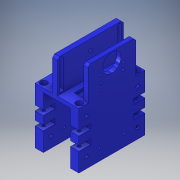
# Autodesk Inventor part: КВ33.044.501 - Каретка оси Y
Saved by Autodesk Inventor 2019 (Build 230136000, 136)
## iProperties
Created: 2019-07-21
Part Number: КВ33.044.501 - Каретка оси Y
Material: Пластик АБС
Document SubType Name: Modeling
Designer: Петров Иван
Density: 1.06 g/cm^3
Appearance: Синий — малярная краска — глянцевая
Mass: 139.056 g
Surface Area: 506.094 cm^2
Volume: 131.185 cm^3
Author: Петров Иван
Autodesk Inventor part; units mm, degrees
(part 1 of 2)
ref_plane "YZ Plane" through (0, 0, 0) normal (1, 0, 0) x (0, 1, 0)
ref_plane "XZ Plane" through (0, 0, 0) normal (0, 1, 0) x (-1, 0, 0)
ref_plane "XY Plane" through (0, 0, 0) normal (0, 0, 1) x (1, 0, 0)
sketch "Эскиз1" plane through (0, 0, 0) normal (1, 0, 0) x (0, 1, 0)
  line L0 (-34, 40) -> (34, 40)
  line L1 (34, 40) -> (34, -40)
  line L2 (34, -40) -> (-34, -40)
  line L3 (-34, -40) -> (-34, 40)
  line L4 (-34, 40) -> (34, -40) construction
  line L5 (34, 40) -> (-34, -40) construction
  line L6 (0, 0) -> (0, 31)
  line L7 (0, 31) -> (21.3, 31)
  line L8 (0, 31) -> (-21.3, 31)
  line L9 (0, 0) -> (0, -31)
  line L10 (0, -31) -> (21.3, -31)
  line L11 (0, -31) -> (-21.3, -31)
  circle A0 centre (21.3, 31) radius 2.1
  circle A1 centre (-21.3, 31) radius 2.1
  circle A2 centre (21.3, -31) radius 2.1
  circle A3 centre (-21.3, -31) radius 2.1
  dimension "d0" = 68
  dimension "d1" = 80
  dimension "d2" = 21.3
  dimension "d3" = 21.3
  dimension "d4" = 31
  dimension "d5" = 31
  dimension "d6" = 21.3
  dimension "d7" = 21.3
  dimension "d8" = 4.2
  dimension "d9" = 4.2
  dimension "d10" = 4.2
  dimension "d11" = 4.2
  constraints: 24 end point, 4 centre point, 4 coincident, 3 horizontal, 3 perpendicular, 2 midpoint, 2 parallel, 2 vertical
  measures "d0" distance of L1.end L2.end
  measures "d1" distance of L0.end L1.end
  measures "d2" distance of L6.end L7.end
  measures "d3" distance of L6.end L8.end
  measures "d4" distance of L6.start L6.end
  measures "d5" distance of L6.start L9.end
  measures "d6" distance of L9.end L10.end
  measures "d7" distance of L9.end L11.end
  measures "d8" diameter of A0
  measures "d9" diameter of A1
  measures "d10" diameter of A2
  measures "d11" diameter of A3
extrude "Выдавливание1" add sketch "Эскиз1" along normal blind 10
sketch "Эскиз2" plane through (10, 0, 0) normal (1, 0, 0) x (0, 0, -1)
  line L0 (-40, 34) -> (-40, -34) projected
  line L1 (-40, 0) -> (-40, 5)
  line L2 (-40, 0) -> (-26, 0)
  line L3 (-26, 0) -> (-26, 11)
  line L4 (-40, 5) -> (-26, 5)
  line L5 (-26, 5) -> (-26, 11)
  line L6 (-26, 11) -> (-40, 11)
  line L7 (-40, 11) -> (-40, 5)
  line L8 (-40, 0) -> (-40, -5)
  line L9 (-26, 0) -> (-26, -11)
  line L10 (-40, -5) -> (-26, -5)
  line L11 (-26, -5) -> (-26, -11)
  line L12 (-26, -11) -> (-40, -11)
  line L13 (-40, -11) -> (-40, -5)
  line L14 (40, -34) -> (40, 34) projected
  line L15 (40, 0) -> (40, 5)
  line L16 (40, 0) -> (26, 0)
  line L17 (26, 0) -> (26, 11)
  line L18 (26, 11) -> (40, 11)
  line L19 (40, 11) -> (40, 5)
  line L20 (40, 5) -> (26, 5)
  line L21 (26, 5) -> (26, 11)
  line L22 (26, 0) -> (26, -11)
  line L23 (40, 0) -> (40, -5)
  line L24 (26, -11) -> (40, -11)
  line L25 (40, -11) -> (40, -5)
  line L26 (40, -5) -> (26, -5)
  line L27 (26, -5) -> (26, -11)
  point P0 (0, 0)
  dimension "d14" = 5
  dimension "d15" = 14
  dimension "d16" = 11
  dimension "d17" = 5
  dimension "d18" = 11
  dimension "d19" = 5
  dimension "d20" = 14
  dimension "d21" = 11
  dimension "d22" = 11
  dimension "d23" = 5
  constraints: 52 end point, 8 parallel, 7 perpendicular, 5 horizontal, 4 point on line, 2 midpoint, 2 vertical
  measures "d14" distance of L1.start L1.end
  measures "d15" distance of L1.start L2.end
  measures "d16" distance of L2.end L3.end
  measures "d17" distance of L1.start L8.end
  measures "d18" distance of L2.end L9.end
  measures "d19" distance of L15.start L15.end
  measures "d20" distance of L15.start L16.end
  measures "d21" distance of L16.end L17.end
  measures "d22" distance of L16.end L22.end
  measures "d23" distance of L15.start L23.end
extrude "Выдавливание2" cut sketch "Эскиз2" against normal blind 10 contours L6 L3 L4 L0 | L10 L9 L12 L0 | L24 L22 L26 L14 | L20 L17 L18 L14
sketch "Эскиз3" plane through (0, 34, 40) normal (0, 1, 0) x (1, 0, 0)
  line L0 (0, 0) -> (10, 0) projected
  line L1 (5, 0) -> (5, 11.1)
  line L2 (0, 11.1) -> (10, 11.1) projected
  circle A0 centre (5, 5.55) radius 1.8
  line L3 (0, 80) -> (10, 80) projected
  line L4 (5, 80) -> (5, 68.9)
  line L5 (0, 68.9) -> (10, 68.9) projected
  circle A1 centre (5, 74.45) radius 1.8
  point P0 (0, 40)
  dimension "d26" = 3.6
  dimension "d29" = 3.6
  constraints: 6 midpoint, 4 end point, 2 centre point
  measures "d26" diameter of A0
  measures "d29" diameter of A1
extrude "Выдавливание3" cut sketch "Эскиз3" against normal through all
sketch "Эскиз4" plane through (0, 34, 40) normal (0, 1, 0) x (1, 0, 0)
  circle A0 centre (5, 5.55) radius 1.8 projected
  circle A1 centre (5, 5.55) radius 4
  circle A2 centre (5, 74.45) radius 1.8 projected
  circle A3 centre (5, 74.45) radius 4
  point P0 (0, 40)
  dimension "d30" = 8
  dimension "d31" = 8
  constraints: 2 centre point, 2 coincident
  measures "d30" diameter of A1
  measures "d31" diameter of A3
extrude "Выдавливание4" cut sketch "Эскиз4" against normal blind 10
sketch "Эскиз5" plane through (10, 0, 0) normal (1, 0, 0) x (0, 0, -1)
  line L0 (0, 0) -> (0, 18)
  line L1 (0, 18) -> (0, 20)
  line L2 (0, 20) -> (-15, 20)
  line L3 (-15, 20) -> (15, 20)
  circle A0 centre (-15, 20) radius 1.5
  circle A1 centre (15, 20) radius 1.5
  line L4 (0, 0) -> (6.6954, 0)
  line L5 (0, -18) -> (0, -20)
  line L6 (0, -20) -> (-15, -20)
  line L7 (-15, -20) -> (15, -20)
  circle A2 centre (-15, -20) radius 1.5
  circle A3 centre (15, -20) radius 1.5
  dimension "d34" = 18
  dimension "d35" = 2
  dimension "d36" = 15
  dimension "d37" = 30
  dimension "d38" = 3
  dimension "d39" = 3
  constraints: 16 end point, 6 symmetric about line, 4 centre point, 4 coincident, 3 point on line, 2 horizontal, 1 vertical, 2 other
  measures "d34" distance of L0.start L0.end
  measures "d35" distance of L0.end L1.end
  measures "d36" distance of L1.end L2.end
  measures "d37" distance of L2.end L3.end
  measures "d38" diameter of A0
  measures "d39" diameter of A1
extrude "Выдавливание5" cut sketch "Эскиз5" against normal blind 10 contours A2 | A3
sketch "Эскиз6" plane through (10, 0, 0) normal (1, 0, 0) x (0, 0, -1)
  circle A0 centre (15, -20) radius 1.5 projected
  circle A1 centre (-15, -20) radius 1.5 projected
  circle A2 centre (-31, 21.3) radius 2.1 projected
  circle A3 centre (-31, -21.3) radius 2.1 projected
  circle A4 centre (31, 21.3) radius 2.1 projected
  circle A5 centre (31, -21.3) radius 2.1 projected
  line L0 (-40, 11) -> (-26, 11) projected
  line L1 (-26, 11) -> (-26, 5) projected
  line L2 (-26, 5) -> (-40, 5) projected
  line L3 (-40, 5) -> (-40, -5) projected
  line L4 (-40, -5) -> (-26, -5) projected
  line L5 (-26, -5) -> (-26, -11) projected
  line L6 (-26, -11) -> (-40, -11) projected
  line L7 (-40, -11) -> (-40, -34) projected
  line L8 (-40, -34) -> (40, -34) projected
  line L9 (40, -34) -> (40, -11) projected
  line L10 (40, -11) -> (26, -11) projected
  line L11 (26, -11) -> (26, -5) projected
  line L12 (26, -5) -> (40, -5) projected
  line L13 (40, -5) -> (40, 5) projected
  line L14 (40, 5) -> (26, 5) projected
  line L15 (26, 5) -> (26, 11) projected
  line L16 (26, 11) -> (40, 11) projected
  line L17 (40, 11) -> (40, 34) projected
  line L18 (40, 34) -> (-40, 34) projected
  line L19 (-40, 34) -> (-40, 11) projected
  point P0 (0, 0)
sketch "Эскиз8" plane through (0, 0, 0) normal (-1, 0, 0) x (0, 0, 1)
  line L0 (-40, 34) -> (-40, 11) projected
  line L1 (40, 11) -> (40, 34) projected
  line L2 (-40, 34) -> (40, 34)
  line L3 (40, 34) -> (40, 29)
  line L4 (40, 29) -> (-40, 29)
  line L5 (-40, 29) -> (-40, 34)
  point P0 (0, 0)
  dimension "d46" = 5
  constraints: 8 end point, 2 parallel, 1 horizontal, 1 perpendicular, 1 point on line
  measures "d46" distance of L2.end L3.end
extrude "Выдавливание7" add sketch "Эскиз8" along normal blind 33
sketch "Эскиз13" plane through (-33, 0, 0) normal (-1, 0, 0) x (0, 0, 1)
  circle A0 centre (15, -20) radius 1.5
  circle A1 centre (-15, -20) radius 1.5
  circle A2 centre (-31, 21.3) radius 2.1
  circle A3 centre (-31, -21.3) radius 2.1
  circle A4 centre (31, 21.3) radius 2.1
  circle A5 centre (31, -21.3) radius 2.1
  line L0 (-40, 11) -> (-26, 11)
  line L1 (-26, 11) -> (-26, 5)
  line L2 (-26, 5) -> (-40, 5)
  line L3 (-40, 5) -> (-40, -5)
  line L4 (-40, -5) -> (-26, -5)
  line L5 (-26, -5) -> (-26, -11)
  line L6 (-26, -11) -> (-40, -11)
  line L7 (-40, -11) -> (-40, -34)
  line L8 (-40, -34) -> (40, -34)
  line L9 (40, -34) -> (40, -11)
  line L10 (40, -11) -> (26, -11)
  line L11 (26, -11) -> (26, -5)
  line L12 (26, -5) -> (40, -5)
  line L13 (40, -5) -> (40, 5)
  line L14 (40, 5) -> (26, 5)
  line L15 (26, 5) -> (26, 11)
  line L16 (26, 11) -> (40, 11)
  line L17 (40, 11) -> (40, 34)
  line L18 (40, 34) -> (-40, 34)
  line L19 (-40, 34) -> (-40, 11)
  point P0 (0, 0)
  point P1 (0, 0)
  constraints: 40 end point, 6 centre point
extrude "Выдавливание11" add sketch "Эскиз13" along normal blind 10
sketch "Эскиз14" plane through (10, 34, 40) normal (0, 1, 0) x (1, 0, 0)
  line L0 (0, 80) -> (-53, 80) projected
  line L1 (-26.5, 80) -> (-26.5, 69.4857)
  circle A0 centre (-5, 5.55) radius 4 projected
  circle A1 centre (-5, 74.45) radius 4 projected
  line L2 (0, 0) -> (-53, 0) projected
  line L3 (0, 80) -> (0, 0) projected
  line L4 (0, 80) -> (-53, 80) projected
  line L5 (-53, 0) -> (-53, 80) projected
  circle A2 centre (-5, 5.55) radius 1.8 projected
  circle A3 centre (-5, 74.45) radius 1.8 projected
  circle A4 centre (-48, 5.55) radius 1.8
  circle A5 centre (-48, 74.45) radius 1.8
  point P0 (-10, 40)
  constraints: 2 centre point, 2 end point, 2 symmetric about line, 1 midpoint, 1 vertical, 2 other
extrude "Выдавливание12" cut sketch "Эскиз14" against normal through all contours A4 | A5
sketch "Эскиз15" plane through (10, 34, 40) normal (0, 1, 0) x (1, 0, 0)
  circle A0 centre (-48, 74.45) radius 1.8 projected
  circle A1 centre (-48, 74.45) radius 4
  circle A2 centre (-48, 5.55) radius 1.8 projected
  circle A3 centre (-48, 5.55) radius 4
  point P0 (-10, 40)
  dimension "d65" = 8
  dimension "d66" = 8
  constraints: 2 centre point, 2 coincident
  measures "d65" diameter of A1
  measures "d66" diameter of A3
extrude "Выдавливание13" cut sketch "Эскиз15" against normal blind 20
sketch "Эскиз16" plane through (10, 34, 40) normal (0, 1, 0) x (1, 0, 0)
  circle A0 centre (-48, 74.45) radius 4 projected
  circle A1 centre (-48, 5.55) radius 4 projected
  circle A2 centre (-5, 5.55) radius 4 projected
  circle A3 centre (-5, 74.45) radius 4 projected
  line L0 (0, 0) -> (-53, 0) projected
  line L1 (0, 80) -> (0, 0) projected
  line L2 (0, 80) -> (-53, 80) projected
  line L3 (-53, 0) -> (-53, 80) projected
  point P0 (-10, 40)
sketch "Эскиз17" plane through (-33, -34, -40) normal (0, -1, 0) x (1, 0, 0)
  circle A0 centre (-5, 5.55) radius 4
  circle A1 centre (-5, 74.45) radius 4
  circle A2 centre (-5, 5.55) radius 1.8 projected
  line L0 (-5, 5.55) -> (-5, 18.1127)
  circle A3 centre (38, 74.45) radius 4
  circle A4 centre (38, 5.55) radius 4
  circle A5 centre (-5, 5.55) radius 4
  circle A6 centre (-5, 74.45) radius 4
  line L1 (-10, 0) -> (43, 0)
  line L2 (-10, 80) -> (-10, 0)
  line L3 (-10, 80) -> (43, 80)
  line L4 (43, 0) -> (43, 80)
  circle A7 centre (-5, 5.55) radius 1.8
  point P0 (33, 40)
  point P1 (-10, 40)
  point P2 (0, 40)
  constraints: 10 end point, 7 centre point, 1 symmetric about line, 1 vertical, 3 other
extrude "Выдавливание14" cut sketch "Эскиз17" against normal blind 20 contours A0 | A1 | A3 | A4
sketch "Эскиз25" plane through (10, 34, 40) normal (0, 1, 0) x (1, 0, 0)
  line L0 (-10, 68.9) -> (0, 68.9) projected
  line L1 (-10, 11.1) -> (0, 11.1) projected
  line L2 (-5, 68.9) -> (0, 68.9)
  line L3 (0, 68.9) -> (0, 11.1)
  line L4 (0, 11.1) -> (-5, 11.1)
  line L5 (-5, 11.1) -> (-5, 68.9)
  point P0 (-10, 40)
  constraints: 8 end point, 2 parallel, 1 horizontal, 1 midpoint, 1 perpendicular, 1 point on line
extrude "Выдавливание21" add sketch "Эскиз25" along normal blind 40
sketch "Эскиз26" plane through (10, 0, 0) normal (1, 0, 0) x (0, 0, -1)
  line L0 (-12.6, 44.2) -> (-14.9, 44.2)
  line L1 (-12.6, 44.2) -> (-12.6, 42.8)
  line L2 (-14.9, 42.8) -> (-12.6, 42.8)
  line L3 (-14.9, 36.2) -> (-14.9, 42.8)
  line L4 (-12.6, 36.2) -> (-14.9, 36.2)
  circle A0 centre (0, 62) radius 9.15
  circle A1 centre (0, 62) radius 1.5
  circle A2 centre (8, 26) radius 1.3
  circle A3 centre (13.5, 39.5) radius 1.3
  circle A4 centre (13.5, 31.5) radius 1.3
  circle A5 centre (13.5, 47.5) radius 1.3
  circle A6 centre (13.5, 55.5) radius 1.3
  circle A7 centre (-8, 26) radius 1.3
  circle A8 centre (-13.5, 39.5) radius 1.3
  circle A9 centre (-13.5, 31.5) radius 1.3
  circle A10 centre (-13.5, 47.5) radius 1.3
  circle A11 centre (-13.5, 55.5) radius 1.3
  line L5 (-0.1, 73.0198) -> (-0.1, 72.4796)
  line L6 (-7, 73.0198) -> (-0.1, 73.0198)
  arc A12 (-7, 73.0198) -> (-7.75, 72.9686) centre (-7, 67.5) ccw
  line L7 (-7.75, 70.5) -> (-7.75, 72.9686)
  arc A13 (-9.5, 68.75) -> (-7.75, 70.5) centre (-9.5, 70.5) ccw
  line L8 (-10, 68.75) -> (-9.5, 68.75)
  line L9 (-10, 31.1937) -> (-10, 68.75)
  arc A14 (-10, 31.1937) -> (-9.6078, 30.5055) centre (-9.2, 31.1937) ccw
  arc A15 (-9.6078, 30.5055) -> (-8.9945, 29.8922) centre (-10.5, 29) ccw
  arc A16 (-8.9945, 29.8922) -> (-8.3063, 29.5) centre (-8.3063, 30.3) ccw
  line L10 (8.3063, 29.5) -> (-8.3063, 29.5)
  arc A17 (8.3063, 29.5) -> (8.9945, 29.8922) centre (8.3063, 30.3) ccw
  arc A18 (9.6078, 30.5055) -> (8.9945, 29.8922) centre (10.5, 29) ccw
  arc A19 (8.9945, 29.8922) -> (9.6078, 30.5055) centre (10.5, 29) ccw
  line L11 (-11.3229, 68.75) -> (-10, 68.75)
  arc A20 (-11.3229, 68.75) -> (-11.5, 67.4989) centre (-6.9922, 67.4989) ccw
  line L12 (-11.5, 67.4989) -> (-11.5, 60)
  line L13 (-12.6, 60) -> (-11.5, 60)
  line L14 (-12.6, 58.8) -> (-12.6, 60)
  line L15 (-14.9, 58.8) -> (-12.6, 58.8)
  line L16 (-14.9, 52.2) -> (-14.9, 58.8)
  line L17 (-12.6, 52.2) -> (-14.9, 52.2)
  line L18 (-12.6, 50.8) -> (-12.6, 52.2)
  line L19 (-14.9, 50.8) -> (-12.6, 50.8)
  line L20 (-14.9, 44.2) -> (-14.9, 50.8)
  line L21 (-12.6, 44.2) -> (-14.9, 44.2)
  line L22 (-12.6, 42.8) -> (-12.6, 44.2)
  line L23 (-14.9, 42.8) -> (-12.6, 42.8)
  line L24 (-14.9, 36.2) -> (-14.9, 42.8)
  line L25 (-12.6, 36.2) -> (-14.9, 36.2)
  line L26 (-12.6, 34.8) -> (-12.6, 36.2)
  line L27 (-14.9, 34.8) -> (-12.6, 34.8)
  line L28 (-14.9, 28.2) -> (-14.9, 34.8)
  line L29 (-12.6, 28.2) -> (-14.9, 28.2)
  line L30 (-12.6, 26.9802) -> (-12.6, 28.2)
  arc A21 (-12.6, 26.9802) -> (-12.5198, 26.9) centre (-11.5, 28) ccw
  line L31 (-11.3, 26.9) -> (-12.5198, 26.9)
  line L32 (-11.3, 24.6) -> (-11.3, 26.9)
  line L33 (-4.7, 24.6) -> (-11.3, 24.6)
  line L34 (-4.7, 26.9) -> (-4.7, 24.6)
  line L35 (4.7, 26.9) -> (-4.7, 26.9)
  line L36 (4.7, 24.6) -> (4.7, 26.9)
  line L37 (11.3, 24.6) -> (4.7, 24.6)
  line L38 (11.3, 26.9) -> (11.3, 24.6)
  line L39 (12.5198, 26.9) -> (11.3, 26.9)
  arc A22 (12.5198, 26.9) -> (12.6, 26.9802) centre (11.5, 28) ccw
  line L40 (12.6, 28.2) -> (12.6, 26.9802)
  line L41 (14.9, 28.2) -> (12.6, 28.2)
  line L42 (14.9, 34.8) -> (14.9, 28.2)
  line L43 (12.6, 34.8) -> (14.9, 34.8)
  line L44 (12.6, 36.2) -> (12.6, 34.8)
  line L45 (14.9, 36.2) -> (12.6, 36.2)
  line L46 (14.9, 42.8) -> (14.9, 36.2)
  line L47 (12.6, 42.8) -> (14.9, 42.8)
  line L48 (12.6, 44.2) -> (12.6, 42.8)
  line L49 (14.9, 44.2) -> (12.6, 44.2)
  line L50 (14.9, 50.8) -> (14.9, 44.2)
  line L51 (12.6, 50.8) -> (14.9, 50.8)
  line L52 (12.6, 52.2) -> (12.6, 50.8)
  line L53 (14.9, 52.2) -> (12.6, 52.2)
  line L54 (14.9, 58.8) -> (14.9, 52.2)
  line L55 (12.6, 58.8) -> (14.9, 58.8)
  line L56 (12.6, 60) -> (12.6, 58.8)
  line L57 (11.5, 60) -> (12.6, 60)
  line L58 (11.5, 67.5) -> (11.5, 60)
  arc A23 (11.5, 67.5) -> (11.3229, 68.75) centre (6.9922, 67.4989) ccw
  line L59 (10, 68.75) -> (11.3229, 68.75)
  line L60 (9.5, 68.75) -> (10, 68.75)
  arc A24 (7.75, 70.5) -> (9.5, 68.75) centre (9.5, 70.5) ccw
  line L61 (7.75, 72.9686) -> (7.75, 70.5)
  arc A25 (7.75, 72.9686) -> (7, 73.0198) centre (7, 67.5) ccw
  line L62 (0.1, 73.0198) -> (7, 73.0198)
  line L63 (0.1, 72.4796) -> (0.1, 73.0198)
  arc A26 (-8.9945, 29.8922) -> (-9.6078, 30.5055) centre (-10.5, 29) ccw
  arc A27 (9.6078, 30.5055) -> (10, 31.1895) centre (9.2, 31.1937) ccw
  line L64 (10, 68.75) -> (10, 31.1895)
  line L65 (0, 0) -> (0, 74)
  line L66 (28.9, 74) -> (-28.9, 74) projected
  line L67 (0, 74) -> (0, 62)
  point P0 (0, 62)
  dimension "d102" = 12
  constraints: 134 end point, 32 point on circle, 28 centre point, 1 midpoint, 1 point on line
  measures "d102" distance of L65.end L67.end
extrude "Выдавливание22" cut sketch "Эскиз26" against normal blind 40 contours A0 L65 A1 | L65 A1 A0 | L65 A1 | A1 L65 | A3 | A5 | A6 | A8 | A10 | A11
sketch "Эскиз29" plane through (-43, 34, -40) normal (0, 1, 0) x (1, 0, 0)
  line L0 (43, -11.1) -> (53, -11.1) projected
  line L1 (48, -11.1) -> (48, -68.9) projected
  line L2 (48, -11.1) -> (48, -68.9)
  circle A0 centre (40.9968, -58.9777) radius 1.5
  line L3 (33.923, -34.3302) -> (33.923, -66.4777)
  line L4 (33.923, -66.4777) -> (47.9968, -66.4777)
  line L5 (47.9968, -66.4777) -> (47.9968, -34.3302)
  line L6 (47.9968, -34.3302) -> (33.923, -34.3302)
  point P0 (43, -40)
  point P1 (40.9968, -50.4777)
  constraints: 10 end point, 1 centre point, 1 collinear, 1 midpoint
extrude "Выдавливание23" cut sketch "Эскиз29" against normal blind 4 contours A0 | L6 L5 L4 L3
sketch "Эскиз30" plane through (-43, 34, -40) normal (0, 1, 0) x (1, 0, 0)
  line L0 (43, -11.1) -> (53, -11.1) projected
  line L1 (48, -11.1) -> (28.26, -11.1)
  line L2 (43, 0) -> (10, 0) projected
  line L3 (53, -80) -> (0, -80) projected
  line L4 (27, 0) -> (21, 0)
  line L5 (21, 0) -> (21, -80)
  line L6 (21, -80) -> (27, -80)
  line L7 (27, -80) -> (27, 0)
  line L8 (48, -11.1) -> (48, -68.9) projected
  point P0 (43, -40)
  dimension "d115" = 19.74
  dimension "d116" = 6
  dimension "d119" = 21
  constraints: 10 end point, 2 parallel, 2 point on line, 1 collinear, 1 horizontal, 1 midpoint, 1 perpendicular
  measures "d115" distance of L1.start L1.end
  measures "d116" distance of L6.end L5.end
  measures "d119" distance between parallel lines of L8 L7
extrude "Выдавливание24" add sketch "Эскиз30" along normal blind 40
sketch "Эскиз31" plane through (-22, 34, -40) normal (-1, 0, 0) x (0, 0, 1)
  circle A0 centre (40, 28) radius 9.15 projected
  circle A1 centre (40, 28) radius 2
  point P0 (40, -34)
  dimension "d120" = 4
  constraints: 1 centre point, 1 coincident
  measures "d120" diameter of A1
extrude "Выдавливание25" cut sketch "Эскиз31" against normal blind 40 contours A1
sketch "Эскиз32" plane through (-16, 34, 40) normal (1, 0, 0) x (0, 0, -1)
  line L0 (0, 0) -> (0, 40) projected
  line L1 (0, 20) -> (5, 20)
  line L2 (5, 3.4608) -> (5, 36.5392) construction
  line L3 (7.1, 3.4608) -> (7.1, 36.5392)
  line L4 (2.9, 36.5392) -> (2.9, 3.4608)
  arc A0 (2.9, 3.4608) -> (7.1, 3.4608) centre (5, 3.4608) ccw
  arc A1 (7.1, 36.5392) -> (2.9, 36.5392) centre (5, 36.5392) ccw
  line L5 (80, 40) -> (0, 40) projected
  line L6 (40, 40) -> (40, 35.6564)
  line L7 (80, 20) -> (75, 20)
  line L8 (75, 3.4608) -> (75, 36.5392) construction
  line L9 (72.9, 3.4608) -> (72.9, 36.5392)
  line L10 (77.1, 36.5392) -> (77.1, 3.4608)
  arc A2 (72.9, 3.4608) -> (77.1, 3.4608) centre (75, 3.4608) ccw
  arc A3 (77.1, 36.5392) -> (72.9, 36.5392) centre (75, 36.5392) ccw
  point P0 (40, -34)
  dimension "d123" = 5
  dimension "d124" = 4.2
  constraints: 22 end point, 8 point on circle, 8 symmetric about line, 4 centre point, 4 tangent, 3 midpoint, 1 horizontal, 1 parallel, 1 perpendicular, 1 vertical, 2 other
  measures "d123" distance of L1.start L1.end
  measures "d124" diameter of A1
extrude "Выдавливание26" cut sketch "Эскиз32" against normal blind 40
sketch "Эскиз33" plane through (10, 0, 0) normal (1, 0, 0) x (0, 0, -1)
  circle A0 centre (0, 62) radius 2 projected
  circle A1 centre (0, 62) radius 11
  point P0 (0, 0)
  dimension "d127" = 22
  constraints: 1 centre point, 1 coincident
  measures "d127" diameter of A1
extrude "Выдавливание27" cut sketch "Эскиз33" against normal blind 6
chamfer "Фаска5" distance 2.75 angle 45 4 edges at (7.5, 74, 28.9) (7.5, 74, -28.9) (-19, 74, 40) (-19, 74, -40)
sketch "Эскиз43" plane through (-43, 34, 40) normal (0, 1, 0) x (1, 0, 0)
  line L0 (0.0943, 0) -> (0.6069, 0)
  line L1 (0.6069, 0) -> (0.6986, 1.434)
  arc A0 (4.89, 1.434) -> (0.6986, 1.434) centre (2.7943, 1.3) ccw
  line L2 (4.89, 1.434) -> (4.9817, 0)
  line L3 (4.9817, 0) -> (9.27, 0)
  arc A1 (9.27, 0) -> (9.3408, 0.0293) centre (9.27, 0.1) ccw
  line L4 (9.3408, 0.0293) -> (9.665, 0.3536)
  arc A2 (10.0186, 0.5) -> (9.665, 0.3536) centre (10.0186, 0) ccw
  line L5 (10.0186, 0.5) -> (19.6943, 0.5)
  arc A3 (19.6943, 0.5) -> (19.7943, 0.6) centre (19.6943, 0.6) ccw
  line L6 (19.7943, 0.6) -> (19.7943, 9.6674)
  arc A4 (19.7943, 9.6674) -> (19.6117, 9.85) centre (19.6943, 9.75) ccw
  line L7 (19.6117, 9.85) -> (16.7686, 9.85)
  arc A5 (16.415, 9.9965) -> (16.7686, 9.85) centre (16.7686, 10.35) ccw
  line L8 (16.415, 9.9965) -> (16.0908, 10.3207)
  arc A6 (16.0908, 10.3207) -> (16.02, 10.35) centre (16.02, 10.25) ccw
  line L9 (16.02, 10.35) -> (13.2686, 10.35)
  arc A7 (13.2686, 10.35) -> (13.1979, 10.3207) centre (13.2686, 10.25) ccw
  line L10 (13.1979, 10.3207) -> (12.8736, 9.9965)
  arc A8 (12.52, 9.85) -> (12.8736, 9.9965) centre (12.52, 10.35) ccw
  line L11 (12.52, 9.85) -> (7.2686, 9.85)
  arc A9 (6.915, 9.9965) -> (7.2686, 9.85) centre (7.2686, 10.35) ccw
  line L12 (6.915, 9.9965) -> (6.5908, 10.3207)
  arc A10 (6.5908, 10.3207) -> (6.52, 10.35) centre (6.52, 10.25) ccw
  line L13 (6.52, 10.35) -> (3.7686, 10.35)
  arc A11 (3.7686, 10.35) -> (3.6979, 10.3207) centre (3.7686, 10.25) ccw
  line L14 (3.6979, 10.3207) -> (3.3736, 9.9965)
  arc A12 (3.02, 9.85) -> (3.3736, 9.9965) centre (3.02, 10.35) ccw
  line L15 (3.02, 9.85) -> (0.0943, 9.85)
  arc A13 (0.0943, 9.85) -> (-0.0057, 9.75) centre (0.0943, 9.75) ccw
  line L16 (-0.0057, 9.75) -> (-0.0057, 0.1)
  arc A14 (-0.0057, 0.1) -> (0.0943, 0) centre (0.0943, 0.1) ccw
  circle A15 centre (5.1443, 7.8) radius 1.25
  circle A16 centre (14.6443, 7.8) radius 1.25
  line L17 (15.8176, 5.55) -> (15.201, 4.25)
  line L18 (15.201, 4.25) -> (15.1843, 4.25)
  line L19 (15.1843, 4.25) -> (14.5843, 5.55)
  line L20 (14.5843, 5.55) -> (14.7111, 5.55)
  line L21 (14.7111, 5.55) -> (14.9033, 5.1334)
  line L22 (14.9033, 5.1334) -> (15.4926, 5.1334)
  line L23 (15.4926, 5.1334) -> (15.6903, 5.55)
  line L24 (15.6903, 5.55) -> (15.8176, 5.55)
  spline S0 degree 3 poles (12.9976, 4.6136) (12.9979, 4.6047) (12.9983, 4.5872) (13.0025, 4.5616) (13.0087, 4.5369) (13.0176, 4.513) (13.0293, 4.4901) (13.0436, 4.4684) (13.0601, 4.4473) (13.0791, 4.4276) (13.1001, 4.4095) (13.1222, 4.3935) (13.1457, 4.3801) (13.1703, 4.3691) (13.196, 4.3605) (13.2229, 4.3545) (13.2508, 4.3508) (13.2699, 4.3503) (13.2797, 4.35) knots 0 0 0 0 0.061965 0.122122 0.180988 0.239933 0.299906 0.359989 0.421776 0.486576 0.551535 0.615018 0.677259 0.73973 0.80305 0.866495 0.931973 1 1 1 1
  spline S1 degree 3 poles (13.2797, 4.35) (13.2898, 4.3503) (13.3098, 4.3508) (13.3391, 4.3545) (13.3671, 4.3607) (13.3938, 4.3694) (13.4192, 4.3803) (13.4433, 4.3939) (13.466, 4.4102) (13.4873, 4.4286) (13.5069, 4.4492) (13.5242, 4.472) (13.5393, 4.4969) (13.5524, 4.5236) (13.5631, 4.5524) (13.5713, 4.5832) (13.5777, 4.6159) (13.5799, 4.6384) (13.581, 4.65) knots 0 0 0 0 0.064439 0.126547 0.186887 0.245878 0.304041 0.362191 0.420976 0.48066 0.5406 0.600689 0.661936 0.724443 0.789038 0.856314 0.926352 1 1 1 1
  line L25 (13.581, 4.65) -> (13.6976, 4.65)
  spline S2 degree 3 poles (13.6976, 4.65) (13.6969, 4.6345) (13.6954, 4.6041) (13.6884, 4.5598) (13.6784, 4.5175) (13.6642, 4.4774) (13.6467, 4.4393) (13.6256, 4.4032) (13.6006, 4.3694) (13.5723, 4.3382) (13.5416, 4.3095) (13.5084, 4.2848) (13.4736, 4.2638) (13.4371, 4.2464) (13.3987, 4.2332) (13.3586, 4.2235) (13.3167, 4.2176) (13.2882, 4.217) (13.2737, 4.2167) knots 0 0 0 0 0.068791 0.135103 0.198979 0.261904 0.323495 0.385195 0.446969 0.509765 0.572251 0.633405 0.693251 0.752583 0.812579 0.873275 0.93555 1 1 1 1
  spline S3 degree 3 poles (13.2737, 4.2167) (13.2594, 4.217) (13.2314, 4.2177) (13.1905, 4.2233) (13.1516, 4.2321) (13.1147, 4.2445) (13.0802, 4.2611) (13.0477, 4.2811) (13.0169, 4.3042) (12.9892, 4.3314) (12.9638, 4.3605) (12.9418, 4.3915) (12.923, 4.4235) (12.9074, 4.4568) (12.8958, 4.4917) (12.8871, 4.5276) (12.8821, 4.565) (12.8814, 4.5903) (12.881, 4.6031) knots 0 0 0 0 0.069475 0.136517 0.200789 0.26383 0.325735 0.387291 0.449509 0.512968 0.576275 0.63758 0.697903 0.757172 0.816599 0.876653 0.93729 1 1 1 1
  spline S4 degree 3 poles (12.881, 4.6031) (12.8816, 4.6213) (12.8829, 4.6571) (12.8935, 4.7099) (12.9102, 4.761) (12.9302, 4.8021) (12.9505, 4.8353) (12.9687, 4.8626) (12.99, 4.8919) (13.0148, 4.9233) (13.0425, 4.9569) (13.0733, 4.9928) (13.1075, 5.0305) (13.1316, 5.0562) (13.144, 5.0696) knots 0 0 0 0 0.098702 0.195672 0.292422 0.391343 0.444462 0.504229 0.570352 0.642546 0.722288 0.807921 0.90047 1 1 1 1
  line L26 (13.144, 5.0696) -> (13.4693, 5.4167)
  line L27 (13.4693, 5.4167) -> (12.8643, 5.4167)
  line L28 (12.8643, 5.4167) -> (12.8643, 5.55)
  line L29 (12.8643, 5.55) -> (13.7476, 5.55)
  line L30 (13.7476, 5.55) -> (13.2435, 5.012)
  spline S5 degree 3 poles (13.2435, 5.012) (13.2312, 4.9992) (13.2076, 4.9746) (13.1743, 4.9386) (13.1443, 4.9053) (13.1176, 4.8746) (13.0946, 4.8462) (13.0742, 4.8208) (13.0579, 4.7975) (13.0402, 4.7705) (13.023, 4.7375) (13.0083, 4.6972) (12.9993, 4.6557) (12.9982, 4.6277) (12.9976, 4.6136) knots 0 0 0 0 0.110803 0.212829 0.306101 0.390647 0.466924 0.534481 0.593587 0.644557 0.7362 0.825024 0.911986 1 1 1 1
  line L31 (12.4876, 4.9) -> (12.3543, 4.25)
  line L32 (12.3543, 4.25) -> (11.821, 4.25)
  line L33 (11.821, 4.25) -> (11.821, 4.3834)
  line L34 (11.821, 4.3834) -> (12.2632, 4.3834)
  line L35 (12.2632, 4.3834) -> (12.3332, 4.7253)
  spline S6 degree 3 poles (12.3332, 4.7253) (12.3195, 4.7215) (12.2928, 4.7141) (12.2534, 4.7059) (12.2161, 4.701) (12.1918, 4.7003) (12.1801, 4.7) knots 0 0 0 0 0.275068 0.532901 0.773973 1 1 1 1
  spline S7 degree 3 poles (12.1801, 4.7) (12.1656, 4.7003) (12.137, 4.701) (12.0953, 4.7069) (12.0554, 4.7162) (12.0175, 4.7293) (11.9815, 4.7459) (11.9478, 4.7668) (11.9158, 4.7911) (11.8861, 4.8191) (11.8592, 4.8499) (11.8355, 4.883) (11.8154, 4.9181) (11.7992, 4.9556) (11.7863, 4.9949) (11.7777, 5.0366) (11.7719, 5.0802) (11.7713, 5.1101) (11.771, 5.1253) knots 0 0 0 0 0.065808 0.129394 0.190894 0.251281 0.310815 0.370371 0.430768 0.492881 0.555104 0.616067 0.677256 0.73826 0.800762 0.864778 0.931045 1 1 1 1
  spline S8 degree 3 poles (11.771, 5.1253) (11.7712, 5.1359) (11.7717, 5.1569) (11.7742, 5.1882) (11.779, 5.2188) (11.7855, 5.2487) (11.7938, 5.2779) (11.804, 5.3065) (11.8164, 5.3343) (11.83, 5.3615) (11.8453, 5.3876) (11.8623, 5.412) (11.8803, 5.435) (11.8996, 5.4565) (11.9205, 5.4763) (11.9426, 5.4945) (11.9659, 5.5114) (11.9907, 5.5263) (12.0164, 5.54) (12.0433, 5.5513) (12.071, 5.5614) (12.0997, 5.5694) (12.1295, 5.5757) (12.1603, 5.5799) (12.192, 5.5831) (12.2135, 5.5833) (12.2244, 5.5834) knots 0 0 0 0 0.044014 0.087434 0.130118 0.172554 0.214555 0.256298 0.298438 0.340849 0.382715 0.423924 0.464246 0.504074 0.543862 0.583567 0.623094 0.663229 0.703551 0.743938 0.784541 0.82575 0.867757 0.910745 0.954914 1 1 1 1
  spline S9 degree 3 poles (12.2244, 5.5834) (12.2373, 5.5831) (12.2628, 5.5826) (12.3001, 5.5773) (12.3361, 5.5697) (12.3703, 5.5584) (12.4031, 5.5441) (12.4341, 5.5261) (12.464, 5.5057) (12.4917, 5.4816) (12.5174, 5.4552) (12.5404, 5.4266) (12.5609, 5.3963) (12.5785, 5.364) (12.5935, 5.3299) (12.6054, 5.2938) (12.6149, 5.256) (12.6189, 5.2299) (12.621, 5.2167) knots 0 0 0 0 0.065421 0.128708 0.190236 0.250724 0.310637 0.370766 0.431615 0.493523 0.555883 0.617342 0.678668 0.740711 0.802985 0.866803 0.932347 1 1 1 1
  line L36 (12.621, 5.2167) -> (12.5043, 5.2167)
  spline S10 degree 3 poles (12.5043, 5.2167) (12.5014, 5.2291) (12.4959, 5.2529) (12.4838, 5.2864) (12.469, 5.3162) (12.4514, 5.3428) (12.4304, 5.366) (12.4064, 5.3866) (12.3796, 5.4053) (12.3497, 5.4208) (12.3182, 5.4341) (12.2852, 5.4429) (12.2517, 5.4491) (12.229, 5.4497) (12.2176, 5.45) knots 0 0 0 0 0.094687 0.181994 0.264377 0.34218 0.418618 0.496509 0.577369 0.661511 0.746733 0.831258 0.915206 1 1 1 1
  spline S11 degree 3 poles (12.2176, 5.45) (12.2065, 5.4497) (12.1846, 5.4491) (12.1523, 5.4445) (12.1212, 5.4374) (12.0915, 5.4267) (12.0627, 5.4138) (12.0355, 5.3972) (12.0091, 5.3781) (11.9845, 5.3562) (11.9619, 5.332) (11.9419, 5.3062) (11.9253, 5.2787) (11.9113, 5.2499) (11.9006, 5.2196) (11.893, 5.1878) (11.8886, 5.1546) (11.888, 5.1319) (11.8876, 5.1203) knots 0 0 0 0 0.064207 0.126425 0.18768 0.248216 0.308305 0.369661 0.431699 0.495947 0.559758 0.622295 0.683911 0.745092 0.80674 0.869087 0.93329 1 1 1 1
  spline S12 degree 3 poles (11.8876, 5.1203) (11.8879, 5.1099) (11.8884, 5.0895) (11.8923, 5.0596) (11.8991, 5.0314) (11.9085, 5.0046) (11.9205, 4.9792) (11.9352, 4.9553) (11.9528, 4.9331) (11.9728, 4.9127) (11.9949, 4.8938) (12.0192, 4.8777) (12.0453, 4.8641) (12.0728, 4.8525) (12.1025, 4.8441) (12.1338, 4.8378) (12.1669, 4.8341) (12.1895, 4.8336) (12.2012, 4.8334) knots 0 0 0 0 0.065351 0.127916 0.18836 0.247216 0.30563 0.36377 0.422661 0.482687 0.5433 0.604118 0.664965 0.727413 0.791468 0.858055 0.927037 1 1 1 1
  spline S13 degree 3 poles (12.2012, 4.8334) (12.2113, 4.8336) (12.2321, 4.834) (12.264, 4.8373) (12.2975, 4.8426) (12.3325, 4.8499) (12.3692, 4.8594) (12.4073, 4.8708) (12.4471, 4.8844) (12.4739, 4.8947) (12.4876, 4.9) knots 0 0 0 0 0.102203 0.211023 0.3251 0.446502 0.573788 0.708901 0.850358 1 1 1 1
  line L37 (9.041, 5.55) -> (8.4243, 4.25)
  line L38 (8.4243, 4.25) -> (8.4076, 4.25)
  line L39 (8.4076, 4.25) -> (7.8076, 5.55)
  line L40 (7.8076, 5.55) -> (7.9345, 5.55)
  line L41 (7.9345, 5.55) -> (8.1267, 5.1334)
  line L42 (8.1267, 5.1334) -> (8.716, 5.1334)
  line L43 (8.716, 5.1334) -> (8.9136, 5.55)
  line L44 (8.9136, 5.55) -> (9.041, 5.55)
  spline S14 degree 3 poles (7.531, 4.8925) (7.5304, 4.8691) (7.5293, 4.8231) (7.5196, 4.7556) (7.5041, 4.6909) (7.482, 4.6291) (7.454, 4.57) (7.4195, 4.514) (7.3788, 4.4607) (7.3322, 4.4109) (7.2811, 4.3654) (7.2263, 4.3254) (7.1681, 4.292) (7.107, 4.2642) (7.0426, 4.2428) (6.9749, 4.2278) (6.9042, 4.2185) (6.856, 4.2173) (6.8315, 4.2167) knots 0 0 0 0 0.064558 0.127014 0.187955 0.248014 0.307748 0.368235 0.42947 0.492743 0.556258 0.618217 0.679655 0.741246 0.803415 0.866815 0.932328 1 1 1 1
  spline S15 degree 3 poles (6.8315, 4.2167) (6.8166, 4.2169) (6.787, 4.2172) (6.7433, 4.2207) (6.7007, 4.2264) (6.6592, 4.2343) (6.6187, 4.244) (6.5794, 4.2567) (6.5411, 4.2712) (6.5041, 4.2879) (6.4684, 4.3066) (6.4342, 4.3272) (6.4017, 4.3496) (6.3707, 4.3736) (6.3417, 4.3998) (6.3139, 4.4273) (6.2882, 4.4571) (6.2723, 4.4781) (6.2643, 4.4886) knots 0 0 0 0 0.068548 0.135683 0.201215 0.265682 0.329267 0.392395 0.45507 0.517127 0.57879 0.63974 0.700192 0.759806 0.819628 0.879355 0.939512 1 1 1 1
  line L45 (6.2643, 4.4886) -> (6.3664, 4.5667)
  spline S16 degree 3 poles (6.3664, 4.5667) (6.3737, 4.558) (6.3881, 4.5408) (6.4114, 4.5166) (6.4357, 4.4939) (6.4609, 4.4726) (6.4876, 4.4535) (6.515, 4.4356) (6.5437, 4.4195) (6.5833, 4.4) (6.6352, 4.3797) (6.7005, 4.3626) (6.7686, 4.3518) (6.8151, 4.3506) (6.8388, 4.35) knots 0 0 0 0 0.063163 0.125475 0.187121 0.248294 0.309295 0.36985 0.430973 0.492456 0.616148 0.740844 0.868183 1 1 1 1
  spline S17 degree 3 poles (6.8388, 4.35) (6.8518, 4.3502) (6.8778, 4.3505) (6.9163, 4.3544) (6.954, 4.3599) (6.9911, 4.3682) (7.0273, 4.3786) (7.063, 4.391) (7.0976, 4.4063) (7.1317, 4.4233) (7.1643, 4.4425) (7.1951, 4.4634) (7.2241, 4.4858) (7.2512, 4.5098) (7.2766, 4.5353) (7.2999, 4.5626) (7.3211, 4.5915) (7.3407, 4.6217) (7.3582, 4.6531) (7.3729, 4.6858) (7.3859, 4.7193) (7.3962, 4.7539) (7.4043, 4.7894) (7.41, 4.8258) (7.4139, 4.8632) (7.4142, 4.8886) (7.4143, 4.9013) knots 0 0 0 0 0.043955 0.087502 0.130463 0.172752 0.215403 0.25765 0.300153 0.343121 0.385925 0.427686 0.468818 0.509492 0.549883 0.58998 0.630405 0.670869 0.711384 0.751627 0.791776 0.832459 0.873319 0.914543 0.956924 1 1 1 1
  spline S18 degree 3 poles (7.4143, 4.9013) (7.4138, 4.9205) (7.4129, 4.9583) (7.4047, 5.0135) (7.3923, 5.0665) (7.3736, 5.1167) (7.3506, 5.165) (7.3216, 5.2104) (7.2879, 5.2536) (7.2492, 5.2937) (7.2067, 5.3303) (7.1611, 5.3625) (7.1125, 5.3894) (7.0615, 5.4117) (7.0076, 5.4289) (6.951, 5.441) (6.8918, 5.4489) (6.8513, 5.4496) (6.8307, 5.45) knots 0 0 0 0 0.064323 0.12629 0.186726 0.246146 0.305576 0.365429 0.426326 0.48884 0.551725 0.613919 0.675484 0.737334 0.800229 0.864502 0.931041 1 1 1 1
  spline S19 degree 3 poles (6.8307, 5.45) (6.808, 5.4494) (6.7634, 5.4482) (6.6978, 5.4377) (6.6351, 5.4207) (6.5752, 5.397) (6.5183, 5.3662) (6.4642, 5.3288) (6.4129, 5.2844) (6.3821, 5.2506) (6.3664, 5.2334) knots 0 0 0 0 0.128515 0.252949 0.374755 0.49594 0.617181 0.740909 0.867811 1 1 1 1
  line L46 (6.3664, 5.2334) -> (6.2643, 5.3107)
  spline S20 degree 3 poles (6.2643, 5.3107) (6.2725, 5.3213) (6.2889, 5.3424) (6.3155, 5.3723) (6.3434, 5.4003) (6.373, 5.4264) (6.4039, 5.4509) (6.4366, 5.4733) (6.4707, 5.4939) (6.5061, 5.5127) (6.5428, 5.5293) (6.5807, 5.5436) (6.6196, 5.5559) (6.6596, 5.5661) (6.7007, 5.574) (6.7428, 5.5792) (6.786, 5.5829) (6.8152, 5.5832) (6.8299, 5.5834) knots 0 0 0 0 0.061674 0.123053 0.183475 0.243727 0.304279 0.364863 0.425946 0.487391 0.54922 0.611144 0.673529 0.736961 0.800785 0.866013 0.932101 1 1 1 1
  spline S21 degree 3 poles (6.8299, 5.5834) (6.8439, 5.5833) (6.8716, 5.5831) (6.9124, 5.5799) (6.9521, 5.5757) (6.9907, 5.5693) (7.0282, 5.5617) (7.0645, 5.5516) (7.0997, 5.5403) (7.1339, 5.5269) (7.167, 5.5119) (7.1989, 5.4949) (7.2296, 5.476) (7.2593, 5.4558) (7.2878, 5.4335) (7.3152, 5.4095) (7.3416, 5.3838) (7.3579, 5.3653) (7.3661, 5.356) knots 0 0 0 0 0.069663 0.13775 0.203917 0.26878 0.332414 0.394754 0.45618 0.516996 0.577396 0.637198 0.696999 0.756756 0.816554 0.876948 0.938132 1 1 1 1
  spline S22 degree 3 poles (7.3661, 5.356) (7.3793, 5.3398) (7.4055, 5.3077) (7.4389, 5.2556) (7.4676, 5.2012) (7.4908, 5.1442) (7.5089, 5.0848) (7.5214, 5.0228) (7.5296, 4.9585) (7.5305, 4.9147) (7.531, 4.8925) knots 0 0 0 0 0.124329 0.247156 0.36878 0.490734 0.613614 0.738958 0.867311 1 1 1 1
  line L47 (4.4583, 4.3) -> (4.6711, 4.3)
  line L48 (4.8587, 5.4) -> (4.4583, 4.3)
  line L49 (4.3587, 5.4) -> (4.8587, 5.4)
  line L50 (3.9583, 4.3) -> (4.3587, 5.4)
  line L51 (3.7455, 4.3) -> (3.9583, 4.3)
  line L52 (4.1458, 5.4) -> (3.7455, 4.3)
  line L53 (3.9458, 5.4) -> (4.1458, 5.4)
  line L54 (4.0186, 5.6) -> (3.9458, 5.4)
  line L55 (5.1443, 5.6) -> (4.0186, 5.6)
  line L56 (4.6711, 4.3) -> (5.1443, 5.6)
  line L57 (9.8343, 5.55) -> (9.851, 5.55)
  line L58 (9.851, 5.55) -> (10.401, 4.25)
  line L59 (10.401, 4.25) -> (10.276, 4.25)
  line L60 (10.276, 4.25) -> (9.8426, 5.2745)
  line L61 (9.8426, 5.2745) -> (9.4093, 4.25)
  line L62 (9.4093, 4.25) -> (9.2843, 4.25)
  line L63 (9.2843, 4.25) -> (9.8343, 5.55)
  spline S23 degree 3 poles (10.6443, 4.9005) (10.6446, 4.9204) (10.645, 4.9592) (10.6475, 5.0158) (10.6523, 5.0693) (10.6583, 5.1197) (10.6666, 5.1669) (10.6769, 5.211) (10.6883, 5.2522) (10.7023, 5.2902) (10.7177, 5.3255) (10.7344, 5.3584) (10.7524, 5.3893) (10.7719, 5.4179) (10.7927, 5.4444) (10.8153, 5.4684) (10.8389, 5.4904) (10.864, 5.5099) (10.8901, 5.527) (10.9168, 5.5423) (10.9446, 5.5547) (10.9728, 5.5653) (11.0018, 5.5734) (11.0316, 5.579) (11.0621, 5.5829) (11.0827, 5.5832) (11.093, 5.5834) knots 0 0 0 0 0.065063 0.126773 0.185516 0.240765 0.29298 0.34225 0.388919 0.432776 0.474628 0.514775 0.553606 0.591426 0.628028 0.663804 0.698984 0.733591 0.767628 0.801208 0.834264 0.866981 0.89972 0.932702 0.966176 1 1 1 1
  spline S24 degree 3 poles (11.093, 5.5834) (11.1033, 5.5832) (11.1235, 5.5828) (11.1534, 5.5793) (11.1825, 5.5736) (11.2109, 5.5657) (11.2386, 5.5559) (11.2654, 5.5432) (11.2915, 5.5286) (11.3168, 5.512) (11.341, 5.4929) (11.3641, 5.4719) (11.3855, 5.4482) (11.4054, 5.4224) (11.4243, 5.3947) (11.4417, 5.3646) (11.4578, 5.3324) (11.4726, 5.2977) (11.4856, 5.2601) (11.4972, 5.2192) (11.5063, 5.1746) (11.5141, 5.1266) (11.5203, 5.0751) (11.5246, 5.02) (11.5273, 4.9614) (11.5275, 4.9212) (11.5276, 4.9005) knots 0 0 0 0 0.033787 0.066622 0.099285 0.131361 0.163585 0.196104 0.228902 0.262158 0.295991 0.330218 0.36506 0.400951 0.43762 0.475708 0.515381 0.556414 0.599765 0.646424 0.696431 0.749782 0.806573 0.867436 0.931887 1 1 1 1
  spline S25 degree 3 poles (11.5276, 4.9005) (11.5275, 4.8797) (11.5273, 4.8392) (11.5247, 4.7803) (11.5203, 4.7249) (11.5143, 4.6732) (11.507, 4.6252) (11.4973, 4.5809) (11.4862, 4.5402) (11.4733, 4.5029) (11.4589, 4.4685) (11.4431, 4.4364) (11.4254, 4.4066) (11.4069, 4.3787) (11.3867, 4.3531) (11.3654, 4.3295) (11.3422, 4.3083) (11.3179, 4.2891) (11.2923, 4.2722) (11.266, 4.2573) (11.239, 4.2446) (11.2111, 4.2346) (11.1826, 4.2264) (11.1534, 4.2207) (11.1235, 4.2172) (11.1033, 4.2169) (11.093, 4.2167) knots 0 0 0 0 0.068595 0.133246 0.194313 0.251279 0.304513 0.354235 0.400481 0.443411 0.484015 0.523252 0.561042 0.5979 0.633518 0.668314 0.702496 0.736685 0.770293 0.803437 0.835913 0.86846 0.900847 0.933467 0.966258 1 1 1 1
  spline S26 degree 3 poles (11.093, 4.2167) (11.0827, 4.2169) (11.0621, 4.2172) (11.0317, 4.2207) (11.002, 4.2264) (10.9731, 4.2346) (10.9449, 4.2447) (10.9174, 4.2573) (10.8906, 4.2721) (10.8648, 4.2894) (10.8399, 4.3087) (10.8163, 4.3305) (10.7941, 4.3547) (10.7731, 4.3808) (10.7538, 4.4095) (10.7353, 4.4403) (10.7189, 4.4736) (10.703, 4.509) (10.6893, 4.5473) (10.6769, 4.5885) (10.6669, 4.6329) (10.6586, 4.6803) (10.6522, 4.731) (10.6475, 4.7848) (10.645, 4.8417) (10.6446, 4.8806) (10.6443, 4.9005) knots 0 0 0 0 0.033788 0.067194 0.099862 0.132567 0.165151 0.197913 0.231319 0.265083 0.299255 0.334399 0.369943 0.406284 0.444064 0.482998 0.523354 0.565537 0.609613 0.656391 0.705885 0.758325 0.813832 0.872795 0.934722 1 1 1 1
  line L64 (16.7943, 4.9) -> (16.661, 4.25)
  line L65 (16.661, 4.25) -> (16.1276, 4.25)
  line L66 (16.1276, 4.25) -> (16.1276, 4.3834)
  line L67 (16.1276, 4.3834) -> (16.5698, 4.3834)
  line L68 (16.5698, 4.3834) -> (16.6399, 4.7253)
  spline S27 degree 3 poles (16.6399, 4.7253) (16.6261, 4.7215) (16.5995, 4.7141) (16.5601, 4.7059) (16.5227, 4.701) (16.4985, 4.7003) (16.4868, 4.7) knots 0 0 0 0 0.275068 0.532901 0.773973 1 1 1 1
  spline S28 degree 3 poles (16.4868, 4.7) (16.4722, 4.7003) (16.4437, 4.701) (16.4019, 4.7069) (16.3621, 4.7162) (16.3242, 4.7293) (16.2882, 4.7459) (16.2545, 4.7668) (16.2225, 4.7911) (16.1928, 4.8191) (16.1658, 4.8499) (16.1422, 4.883) (16.122, 4.9181) (16.1059, 4.9556) (16.0929, 4.9949) (16.0843, 5.0366) (16.0786, 5.0802) (16.078, 5.1101) (16.0776, 5.1253) knots 0 0 0 0 0.065808 0.129394 0.190894 0.251281 0.310815 0.370371 0.430768 0.492881 0.555104 0.616067 0.677256 0.73826 0.800762 0.864778 0.931045 1 1 1 1
  spline S29 degree 3 poles (16.0776, 5.1253) (16.0779, 5.1359) (16.0784, 5.1569) (16.0809, 5.1882) (16.0857, 5.2188) (16.0921, 5.2487) (16.1005, 5.2779) (16.1106, 5.3065) (16.123, 5.3343) (16.1367, 5.3615) (16.152, 5.3876) (16.169, 5.412) (16.1869, 5.435) (16.2063, 5.4565) (16.2271, 5.4763) (16.2493, 5.4945) (16.2726, 5.5114) (16.2974, 5.5263) (16.323, 5.54) (16.35, 5.5513) (16.3777, 5.5614) (16.4064, 5.5694) (16.4361, 5.5757) (16.467, 5.5799) (16.4987, 5.5831) (16.5202, 5.5833) (16.531, 5.5834) knots 0 0 0 0 0.044014 0.087434 0.130118 0.172554 0.214555 0.256298 0.298438 0.340849 0.382715 0.423924 0.464246 0.504074 0.543862 0.583567 0.623094 0.663229 0.703551 0.743938 0.784541 0.82575 0.867757 0.910745 0.954914 1 1 1 1
  spline S30 degree 3 poles (16.531, 5.5834) (16.544, 5.5831) (16.5695, 5.5826) (16.6068, 5.5773) (16.6427, 5.5697) (16.6769, 5.5584) (16.7098, 5.5441) (16.7408, 5.5261) (16.7707, 5.5057) (16.7984, 5.4816) (16.8241, 5.4552) (16.847, 5.4266) (16.8675, 5.3963) (16.8852, 5.364) (16.9002, 5.3299) (16.912, 5.2938) (16.9216, 5.256) (16.9256, 5.2299) (16.9276, 5.2167) knots 0 0 0 0 0.065421 0.128708 0.190236 0.250724 0.310637 0.370766 0.431615 0.493523 0.555883 0.617342 0.678668 0.740711 0.802985 0.866803 0.932347 1 1 1 1
  line L69 (16.9276, 5.2167) -> (16.811, 5.2167)
  spline S31 degree 3 poles (16.811, 5.2167) (16.8081, 5.2291) (16.8026, 5.2529) (16.7905, 5.2864) (16.7757, 5.3162) (16.7581, 5.3428) (16.7371, 5.366) (16.7131, 5.3866) (16.6862, 5.4053) (16.6564, 5.4208) (16.6249, 5.4341) (16.5919, 5.4429) (16.5583, 5.4491) (16.5357, 5.4497) (16.5243, 5.45) knots 0 0 0 0 0.094687 0.181994 0.264377 0.34218 0.418618 0.496509 0.577369 0.661511 0.746733 0.831258 0.915206 1 1 1 1
  spline S32 degree 3 poles (16.5243, 5.45) (16.5131, 5.4497) (16.4912, 5.4491) (16.459, 5.4445) (16.4278, 5.4374) (16.3981, 5.4267) (16.3693, 5.4138) (16.3421, 5.3972) (16.3158, 5.3781) (16.2911, 5.3562) (16.2685, 5.332) (16.2486, 5.3062) (16.2319, 5.2787) (16.2179, 5.2499) (16.2073, 5.2196) (16.1997, 5.1878) (16.1952, 5.1546) (16.1946, 5.1319) (16.1943, 5.1203) knots 0 0 0 0 0.064207 0.126425 0.18768 0.248216 0.308305 0.369661 0.431699 0.495947 0.559758 0.622295 0.683911 0.745092 0.80674 0.869087 0.93329 1 1 1 1
  spline S33 degree 3 poles (16.1943, 5.1203) (16.1946, 5.1099) (16.195, 5.0895) (16.1989, 5.0596) (16.2057, 5.0314) (16.2152, 5.0046) (16.2272, 4.9792) (16.2418, 4.9553) (16.2594, 4.9331) (16.2795, 4.9127) (16.3015, 4.8938) (16.3258, 4.8777) (16.3519, 4.8641) (16.3795, 4.8525) (16.4092, 4.8441) (16.4404, 4.8378) (16.4736, 4.8341) (16.4962, 4.8336) (16.5079, 4.8334) knots 0 0 0 0 0.065351 0.127916 0.18836 0.247216 0.30563 0.36377 0.422661 0.482687 0.5433 0.604118 0.664965 0.727413 0.791468 0.858055 0.927037 1 1 1 1
  spline S34 degree 3 poles (16.5079, 4.8334) (16.5179, 4.8336) (16.5387, 4.834) (16.5706, 4.8373) (16.6042, 4.8426) (16.6392, 4.8499) (16.6758, 4.8594) (16.714, 4.8708) (16.7538, 4.8844) (16.7805, 4.8947) (16.7943, 4.9) knots 0 0 0 0 0.102203 0.211023 0.3251 0.446502 0.573788 0.708901 0.850358 1 1 1 1
  line L70 (0, 80) -> (0, 0) projected
  line L71 (0, 40) -> (8.6448, 40)
  line L72 (0.0943, 80) -> (0.6069, 80)
  line L73 (0.6069, 80) -> (0.6986, 78.566)
  arc A17 (0.6986, 78.566) -> (4.89, 78.566) centre (2.7943, 78.7) ccw
  line L74 (4.89, 78.566) -> (4.9817, 80)
  line L75 (4.9817, 80) -> (9.27, 80)
  arc A18 (9.3408, 79.9707) -> (9.27, 80) centre (9.27, 79.9) ccw
  line L76 (9.3408, 79.9707) -> (9.665, 79.6464)
  arc A19 (9.665, 79.6464) -> (10.0186, 79.5) centre (10.0186, 80) ccw
  line L77 (10.0186, 79.5) -> (19.6943, 79.5)
  arc A20 (19.7943, 79.4) -> (19.6943, 79.5) centre (19.6943, 79.4) ccw
  line L78 (19.7943, 79.4) -> (19.7943, 70.3326)
  arc A21 (19.6117, 70.15) -> (19.7943, 70.3326) centre (19.6943, 70.25) ccw
  line L79 (19.6117, 70.15) -> (16.7686, 70.15)
  arc A22 (16.7686, 70.15) -> (16.415, 70.0035) centre (16.7686, 69.65) ccw
  line L80 (16.415, 70.0035) -> (16.0908, 69.6793)
  arc A23 (16.02, 69.65) -> (16.0908, 69.6793) centre (16.02, 69.75) ccw
  line L81 (16.02, 69.65) -> (13.2686, 69.65)
  arc A24 (13.1979, 69.6793) -> (13.2686, 69.65) centre (13.2686, 69.75) ccw
  line L82 (13.1979, 69.6793) -> (12.8736, 70.0035)
  arc A25 (12.8736, 70.0035) -> (12.52, 70.15) centre (12.52, 69.65) ccw
  line L83 (12.52, 70.15) -> (7.2686, 70.15)
  arc A26 (7.2686, 70.15) -> (6.915, 70.0035) centre (7.2686, 69.65) ccw
  line L84 (6.915, 70.0035) -> (6.5908, 69.6793)
  arc A27 (6.52, 69.65) -> (6.5908, 69.6793) centre (6.52, 69.75) ccw
  line L85 (6.52, 69.65) -> (3.7686, 69.65)
  arc A28 (3.6979, 69.6793) -> (3.7686, 69.65) centre (3.7686, 69.75) ccw
  line L86 (3.6979, 69.6793) -> (3.3736, 70.0035)
  arc A29 (3.3736, 70.0035) -> (3.02, 70.15) centre (3.02, 69.65) ccw
  line L87 (3.02, 70.15) -> (0.0943, 70.15)
  arc A30 (-0.0057, 70.25) -> (0.0943, 70.15) centre (0.0943, 70.25) ccw
  line L88 (-0.0057, 70.25) -> (-0.0057, 79.9)
  arc A31 (0.0943, 80) -> (-0.0057, 79.9) centre (0.0943, 79.9) ccw
  circle A32 centre (5.1443, 72.2) radius 1.25
  circle A33 centre (14.6443, 72.2) radius 1.25
  line L89 (15.8176, 74.45) -> (15.201, 75.75)
  line L90 (15.201, 75.75) -> (15.1843, 75.75)
  line L91 (15.1843, 75.75) -> (14.5843, 74.45)
  line L92 (14.5843, 74.45) -> (14.7111, 74.45)
  line L93 (14.7111, 74.45) -> (14.9033, 74.8666)
  line L94 (14.9033, 74.8666) -> (15.4926, 74.8666)
  line L95 (15.4926, 74.8666) -> (15.6903, 74.45)
  line L96 (15.6903, 74.45) -> (15.8176, 74.45)
  spline S35 degree 3 poles (12.9976, 75.3864) (12.9979, 75.3953) (12.9983, 75.4128) (13.0025, 75.4384) (13.0087, 75.4631) (13.0176, 75.487) (13.0293, 75.5099) (13.0436, 75.5316) (13.0601, 75.5527) (13.0791, 75.5724) (13.1001, 75.5905) (13.1222, 75.6065) (13.1457, 75.6199) (13.1703, 75.6309) (13.196, 75.6395) (13.2229, 75.6455) (13.2508, 75.6492) (13.2699, 75.6497) (13.2797, 75.65) knots 0 0 0 0 0.061965 0.122122 0.180988 0.239933 0.299906 0.359989 0.421776 0.486576 0.551535 0.615018 0.677259 0.73973 0.80305 0.866495 0.931973 1 1 1 1
  spline S36 degree 3 poles (13.2797, 75.65) (13.2898, 75.6497) (13.3098, 75.6492) (13.3391, 75.6455) (13.3671, 75.6393) (13.3938, 75.6306) (13.4192, 75.6197) (13.4433, 75.6061) (13.466, 75.5898) (13.4873, 75.5714) (13.5069, 75.5508) (13.5242, 75.528) (13.5393, 75.5031) (13.5524, 75.4764) (13.5631, 75.4476) (13.5713, 75.4168) (13.5777, 75.3841) (13.5799, 75.3616) (13.581, 75.35) knots 0 0 0 0 0.064439 0.126547 0.186887 0.245878 0.304041 0.362191 0.420976 0.48066 0.5406 0.600689 0.661936 0.724443 0.789038 0.856314 0.926352 1 1 1 1
  line L97 (13.581, 75.35) -> (13.6976, 75.35)
  spline S37 degree 3 poles (13.6976, 75.35) (13.6969, 75.3655) (13.6954, 75.3959) (13.6884, 75.4402) (13.6784, 75.4825) (13.6642, 75.5226) (13.6467, 75.5607) (13.6256, 75.5968) (13.6006, 75.6306) (13.5723, 75.6618) (13.5416, 75.6905) (13.5084, 75.7152) (13.4736, 75.7362) (13.4371, 75.7536) (13.3987, 75.7668) (13.3586, 75.7765) (13.3167, 75.7824) (13.2882, 75.783) (13.2737, 75.7833) knots 0 0 0 0 0.068791 0.135103 0.198979 0.261904 0.323495 0.385195 0.446969 0.509765 0.572251 0.633405 0.693251 0.752583 0.812579 0.873275 0.93555 1 1 1 1
  spline S38 degree 3 poles (13.2737, 75.7833) (13.2594, 75.783) (13.2314, 75.7823) (13.1905, 75.7767) (13.1516, 75.7679) (13.1147, 75.7555) (13.0802, 75.7389) (13.0477, 75.7189) (13.0169, 75.6958) (12.9892, 75.6686) (12.9638, 75.6395) (12.9418, 75.6085) (12.923, 75.5765) (12.9074, 75.5432) (12.8958, 75.5083) (12.8871, 75.4724) (12.8821, 75.435) (12.8814, 75.4097) (12.881, 75.3969) knots 0 0 0 0 0.069475 0.136517 0.200789 0.26383 0.325735 0.387291 0.449509 0.512968 0.576275 0.63758 0.697903 0.757172 0.816599 0.876653 0.93729 1 1 1 1
  spline S39 degree 3 poles (12.881, 75.3969) (12.8816, 75.3787) (12.8829, 75.3429) (12.8935, 75.2901) (12.9102, 75.239) (12.9302, 75.1979) (12.9505, 75.1647) (12.9687, 75.1374) (12.99, 75.1081) (13.0148, 75.0767) (13.0425, 75.0431) (13.0733, 75.0072) (13.1075, 74.9695) (13.1316, 74.9438) (13.144, 74.9304) knots 0 0 0 0 0.098702 0.195672 0.292422 0.391343 0.444462 0.504229 0.570352 0.642546 0.722288 0.807921 0.90047 1 1 1 1
  line L98 (13.144, 74.9304) -> (13.4693, 74.5833)
  line L99 (13.4693, 74.5833) -> (12.8643, 74.5833)
  line L100 (12.8643, 74.5833) -> (12.8643, 74.45)
  line L101 (12.8643, 74.45) -> (13.7476, 74.45)
  line L102 (13.7476, 74.45) -> (13.2435, 74.988)
  spline S40 degree 3 poles (13.2435, 74.988) (13.2312, 75.0008) (13.2076, 75.0254) (13.1743, 75.0614) (13.1443, 75.0947) (13.1176, 75.1254) (13.0946, 75.1538) (13.0742, 75.1792) (13.0579, 75.2025) (13.0402, 75.2295) (13.023, 75.2625) (13.0083, 75.3028) (12.9993, 75.3443) (12.9982, 75.3723) (12.9976, 75.3864) knots 0 0 0 0 0.110803 0.212829 0.306101 0.390647 0.466924 0.534481 0.593587 0.644557 0.7362 0.825024 0.911986 1 1 1 1
  line L103 (12.4876, 75.1) -> (12.3543, 75.75)
  line L104 (12.3543, 75.75) -> (11.821, 75.75)
  line L105 (11.821, 75.75) -> (11.821, 75.6166)
  line L106 (11.821, 75.6166) -> (12.2632, 75.6166)
  line L107 (12.2632, 75.6166) -> (12.3332, 75.2747)
  spline S41 degree 3 poles (12.3332, 75.2747) (12.3195, 75.2785) (12.2928, 75.2859) (12.2534, 75.2941) (12.2161, 75.299) (12.1918, 75.2997) (12.1801, 75.3) knots 0 0 0 0 0.275068 0.532901 0.773973 1 1 1 1
  spline S42 degree 3 poles (12.1801, 75.3) (12.1656, 75.2997) (12.137, 75.299) (12.0953, 75.2931) (12.0554, 75.2838) (12.0175, 75.2707) (11.9815, 75.2541) (11.9478, 75.2332) (11.9158, 75.2089) (11.8861, 75.1809) (11.8592, 75.1501) (11.8355, 75.117) (11.8154, 75.0819) (11.7992, 75.0444) (11.7863, 75.0051) (11.7777, 74.9634) (11.7719, 74.9198) (11.7713, 74.8899) (11.771, 74.8747) knots 0 0 0 0 0.065808 0.129394 0.190894 0.251281 0.310815 0.370371 0.430768 0.492881 0.555104 0.616067 0.677256 0.73826 0.800762 0.864778 0.931045 1 1 1 1
  spline S43 degree 3 poles (11.771, 74.8747) (11.7712, 74.8641) (11.7717, 74.8431) (11.7742, 74.8118) (11.779, 74.7812) (11.7855, 74.7513) (11.7938, 74.7221) (11.804, 74.6935) (11.8164, 74.6657) (11.83, 74.6385) (11.8453, 74.6124) (11.8623, 74.588) (11.8803, 74.565) (11.8996, 74.5435) (11.9205, 74.5237) (11.9426, 74.5055) (11.9659, 74.4886) (11.9907, 74.4737) (12.0164, 74.46) (12.0433, 74.4487) (12.071, 74.4386) (12.0997, 74.4306) (12.1295, 74.4243) (12.1603, 74.4201) (12.192, 74.4169) (12.2135, 74.4167) (12.2244, 74.4166) knots 0 0 0 0 0.044014 0.087434 0.130118 0.172554 0.214555 0.256298 0.298438 0.340849 0.382715 0.423924 0.464246 0.504074 0.543862 0.583567 0.623094 0.663229 0.703551 0.743938 0.784541 0.82575 0.867757 0.910745 0.954914 1 1 1 1
  spline S44 degree 3 poles (12.2244, 74.4166) (12.2373, 74.4169) (12.2628, 74.4174) (12.3001, 74.4227) (12.3361, 74.4303) (12.3703, 74.4416) (12.4031, 74.4559) (12.4341, 74.4739) (12.464, 74.4943) (12.4917, 74.5184) (12.5174, 74.5448) (12.5404, 74.5734) (12.5609, 74.6037) (12.5785, 74.636) (12.5935, 74.6701) (12.6054, 74.7062) (12.6149, 74.744) (12.6189, 74.7701) (12.621, 74.7833) knots 0 0 0 0 0.065421 0.128708 0.190236 0.250724 0.310637 0.370766 0.431615 0.493523 0.555883 0.617342 0.678668 0.740711 0.802985 0.866803 0.932347 1 1 1 1